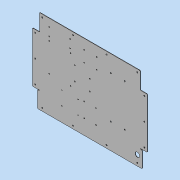
# Autodesk Inventor part: Board_Mount_Flat
Saved by Autodesk Inventor 2020 (Build 240168000, 168)
## iProperties
Created: 2021-06-14
Part Number: Board_Mount_Flat
Material: Generic
Document SubType Name: Modeling
Designer: magnarecta
Density: 1 g/cm^3
Appearance: Default
Author: magnarecta
Autodesk Inventor part; units mm, degrees
ref_plane "YZ Plane" through (0, 0, 0) normal (1, 0, 0) x (0, 1, 0)
ref_plane "XZ Plane" through (0, 0, 0) normal (0, 1, 0) x (-1, 0, 0)
ref_plane "XY Plane" through (0, 0, 0) normal (0, 0, 1) x (1, 0, 0)
sketch "スケッチ1" plane through (0, 0, 0) normal (0, 0, 1) x (1, 0, 0)
  circle A0 centre (380.0191, 230.2191) radius 2.25
  circle A1 centre (380.0191, 70.2191) radius 2.25
  circle A2 centre (380.0191, 150.2191) radius 2.25
  circle A3 centre (124.8, 290.4382) radius 2.25
  circle A4 centre (14.8, 290.4382) radius 2.25
  circle A5 centre (354.8, 290.4382) radius 2.25
  circle A6 centre (244.8, 290.4382) radius 2.25
  circle A7 centre (259.8, 240.2191) radius 2.25
  circle A8 centre (259.8, 90.2191) radius 2.25
  circle A9 centre (309.8, 90.2191) radius 2.25
  circle A10 centre (309.8, 240.2191) radius 2.25
  circle A11 centre (116.1, 128.3691) radius 1.75
  circle A12 centre (39.8, 230.2191) radius 1.75
  circle A13 centre (116.1, 230.2191) radius 1.75
  circle A14 centre (39.8, 128.3691) radius 1.75
  circle A15 centre (131.1, 150.2191) radius 1.75
  circle A16 centre (131.1, 200.2191) radius 1.75
  circle A17 centre (164.8, 105.2191) radius 1.75
  circle A18 centre (206.8, 53.2191) radius 1.75
  circle A19 centre (206.8, 105.2191) radius 1.75
  circle A20 centre (164.8, 53.2191) radius 1.75
  circle A21 centre (209.4, 265.2191) radius 1.75
  circle A22 centre (164.8, 225.4191) radius 1.75
  circle A23 centre (164.8, 265.2191) radius 1.75
  circle A24 centre (209.4, 225.4191) radius 1.75
  circle A25 centre (84.8, 51.2191) radius 1.4
  circle A26 centre (142.8, 51.2191) radius 1.4
  circle A27 centre (142.8, 100.2191) radius 1.4
  circle A28 centre (84.8, 100.2191) radius 1.4
  circle A29 centre (39.8, 273.2191) radius 1.75
  circle A30 centre (114, 244.0191) radius 1.75
  circle A31 centre (114, 273.2191) radius 1.75
  circle A32 centre (39.8, 244.0191) radius 1.75
  circle A33 centre (184.8, 146.1191) radius 1.75
  circle A34 centre (184.8, 185.2191) radius 1.75
  circle A35 centre (354.8, 35.2191) radius 8.25
  circle A36 centre (-10.4191, 150.2191) radius 2.25
  circle A37 centre (-10.4191, 70.2191) radius 2.25
  circle A38 centre (-10.4191, 230.2191) radius 2.25
  circle A39 centre (244.8, 10) radius 2.25
  circle A40 centre (354.8, 10) radius 2.25
  circle A41 centre (14.8, 10) radius 2.25
  circle A42 centre (124.8, 10) radius 2.25
  arc A43 (-2, 2) -> (0, 0) centre (0, 2) ccw
  line L0 (369.6, 0) -> (0, 0)
  arc A44 (369.6, 0) -> (371.6, 2) centre (369.6, 2) ccw
  line L1 (371.6, 2) -> (371.6, 56.2191)
  arc A45 (371.6, 56.2191) -> (369.6, 58.2191) centre (369.6, 56.2191) ccw
  line L2 (369.6, 58.2191) -> (365.6, 58.2191)
  line L3 (365.6, 58.2191) -> (365.6, 60.2191)
  line L4 (365.6, 60.2191) -> (388.0191, 60.2191)
  arc A46 (388.0191, 60.2191) -> (390.0191, 62.2191) centre (388.0191, 62.2191) ccw
  line L5 (390.0191, 238.2191) -> (390.0191, 62.2191)
  arc A47 (390.0191, 238.2191) -> (388.0191, 240.2191) centre (388.0191, 238.2191) ccw
  line L6 (388.0191, 240.2191) -> (366.8, 240.2191)
  arc A48 (364.8, 242.2191) -> (366.8, 240.2191) centre (366.8, 242.2191) ccw
  line L7 (364.8, 242.2191) -> (364.8, 298.4382)
  arc A49 (364.8, 298.4382) -> (362.8, 300.4382) centre (362.8, 298.4382) ccw
  line L8 (6.8, 300.4382) -> (362.8, 300.4382)
  arc A50 (6.8, 300.4382) -> (4.8, 298.4382) centre (6.8, 298.4382) ccw
  line L9 (4.8, 298.4382) -> (4.8, 242.2191)
  arc A51 (2.8, 240.2191) -> (4.8, 242.2191) centre (2.8, 242.2191) ccw
  line L10 (2.8, 240.2191) -> (-18.4191, 240.2191)
  arc A52 (-18.4191, 240.2191) -> (-20.4191, 238.2191) centre (-18.4191, 238.2191) ccw
  line L11 (-20.4191, 62.2191) -> (-20.4191, 238.2191)
  arc A53 (-20.4191, 62.2191) -> (-18.4191, 60.2191) centre (-18.4191, 62.2191) ccw
  line L12 (-18.4191, 60.2191) -> (4, 60.2191)
  line L13 (4, 60.2191) -> (4, 58.2191)
  line L14 (4, 58.2191) -> (0, 58.2191)
  arc A54 (0, 58.2191) -> (-2, 56.2191) centre (0, 56.2191) ccw
  line L15 (-2, 56.2191) -> (-2, 2)
  constraints: 55 centre point, 32 end point, 24 point on circle
extrude "押し出し1" add sketch "スケッチ1" along normal blind 1.6
